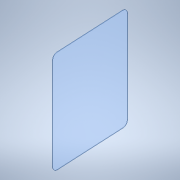
# Autodesk Inventor part: Ventanas
Saved by Autodesk Inventor 2021 (Build 250183000, 183)
## iProperties
Created: 2021-06-03
Part Number: Ventanas
Material: Genérico
Document SubType Name: Modeling
Designer: Mecatronica
Density: 1 g/cm^3
Appearance: Azul - Cristalera
Author: Mecatronica
Autodesk Inventor part; units mm, degrees
ref_plane "YZ Plane" through (0, 0, 0) normal (1, 0, 0) x (0, 1, 0)
ref_plane "XZ Plane" through (0, 0, 0) normal (0, 1, 0) x (-1, 0, 0)
ref_plane "XY Plane" through (0, 0, 0) normal (0, 0, 1) x (1, 0, 0)
sketch "Boceto1" plane through (0, 0, 0) normal (1, 0, 0) x (0, 1, 0)
  line L0 (-522.3171, 332.4506) -> (-488.1102, -337.5494)
  line L1 (561.6295, -332.4506) -> (527.4226, 337.5494)
  line L2 (-472.3821, 385) -> (477.4876, 385)
  line L3 (-438.1752, -385) -> (511.6946, -385)
  arc A0 (-472.3821, 385) -> (-522.3171, 332.4506) centre (-472.3821, 335) ccw
  arc A1 (-488.1102, -337.5494) -> (-438.1752, -385) centre (-438.1752, -335) ccw
  arc A2 (511.6946, -385) -> (561.6295, -332.4506) centre (511.6946, -335) ccw
  arc A3 (527.4226, 337.5494) -> (477.4876, 385) centre (477.4876, 335) ccw
  point P0 (0, 0)
  point P1 (-525, 385)
  point P2 (525, 385)
  point P3 (-485.6876, -385)
  point P4 (564.3124, -385)
  dimension "d17" = 1050
  dimension "d19" = 1050
  dimension "d20" = 770
  dimension "d21" = 385
  dimension "d22" = 525
  dimension "d23" = 50
  dimension "d24" = 50
  constraints: 8 end point, 8 point on circle, 8 point on line, 8 tangent, 4 centre point, 2 equal radius, 1 horizontal
  measures "d17" distance of point (-525, 385) point (525, 385)
  measures "d19" distance of point (-485.688, -385) point (564.312, -385)
  measures "d20" distance between parallel lines of L3 L2
  measures "d21" distance from line of point (0, 0) L2
  measures "d22" horizontal distance of point (0, 0) point (-525, 385)
  measures "d23" radius of A0
  measures "d24" radius of A1
extrude "Extrusión1" add sketch "Boceto1" along normal blind 5
equation "\"d19\" = d17"
equation "\"d21\" = 0.5 * d20"
equation "\"d22\" = 0.5 * d19"
